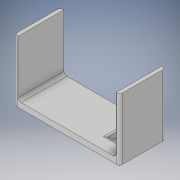
# Autodesk Inventor part: switch mount
Saved by Autodesk Inventor 2017 (Build 210142000, 142)
## iProperties
Created: 2017-11-26
Part Number: switch mount
Material: Generic
Document SubType Name: Modeling
Designer: Mitch
Density: 1 g/cm^3
Appearance: Default
Author: Mitch
Autodesk Inventor part; units mm, degrees
ref_plane "YZ Plane" through (0, 0, 0) normal (1, 0, 0) x (0, 1, 0)
ref_plane "XZ Plane" through (0, 0, 0) normal (0, 1, 0) x (-1, 0, 0)
ref_plane "XY Plane" through (0, 0, 0) normal (0, 0, 1) x (1, 0, 0)
sketch "Sketch1" plane through (0, 0, 0) normal (0, 1, 0) x (-1, 0, 0)
  line L0 (0, 0) -> (57.023, 0)
  line L1 (57.023, 0) -> (57.023, -24.765)
  line L2 (57.023, -24.765) -> (0, -24.765)
  line L3 (0, -24.765) -> (0, 0)
  dimension "d0" = 57.023
  dimension "d1" = 24.765
  constraints: 8 end point, 2 parallel, 1 horizontal, 1 perpendicular
  measures "d0" distance of L1.end L2.end
  measures "d1" distance of L0.end L1.end
extrude "Extrusion1" add sketch "Sketch1" along normal blind 3.175
sketch "Sketch3" plane through (0, 0, 0) normal (0, -1, 0) x (1, 0, 0)
  line L0 (-3.175, -3.175) -> (-15.113, -3.175)
  line L1 (-15.113, -3.175) -> (-15.113, -21.59)
  line L2 (-15.113, -21.59) -> (-3.175, -21.59)
  line L3 (-3.175, -21.59) -> (-3.175, -3.175)
  line L4 (0, -24.765) -> (0, 0) projected
  line L5 (-57.023, 0) -> (0, 0) projected
  dimension "d18" = 18.415
  dimension "d19" = 11.938
  dimension "d20" = 3.175
  dimension "d21" = 3.175
  constraints: 8 end point, 2 parallel, 1 horizontal, 1 perpendicular
  measures "d18" distance of L2.end L0.start
  measures "d19" distance of L1.end L2.end
  measures "d20" distance between parallel lines of L4 L3
  measures "d21" distance between parallel lines of L5 L0
extrude "Extrusion3" add sketch "Sketch3" along normal blind 2.921
fillet "Fillet2" radius 1.5875 4 edges at (0, 1.5875, -24.765) (0, 1.5875, 0) (-57.023, 1.5875, 0) (-57.023, 1.5875, -24.765)
hole "Hole2" at (-9.144, -2.921, -12.3825) direction (0, 1, 0) diameter 10.16 depth 25.4
sketch "Sketch4" plane through (0, 3.175, 0) normal (0, 1, 0) x (1, 0, 0)
  line L0 (-3.8735, 17.653) -> (-14.4145, 17.653)
  line L1 (-14.4145, 17.653) -> (-14.4145, 7.112)
  line L2 (-14.4145, 7.112) -> (-3.8735, 7.112)
  line L3 (-3.8735, 7.112) -> (-3.8735, 17.653)
  line L4 (-1.5875, 24.765) -> (-55.4355, 24.765) projected
  line L5 (0, 1.5875) -> (0, 23.1775) projected
  point P0 (0, 0)
  dimension "d34" = 10.541
  dimension "d35" = 10.541
  dimension "d36" = 7.112
  dimension "d37" = 3.8735
  constraints: 8 end point, 2 parallel, 1 horizontal, 1 perpendicular
  measures "d34" distance of L2.end L1.end
  measures "d35" distance of L1.end L0.end
  measures "d36" distance between parallel lines of L4 L0
  measures "d37" distance between parallel lines of L5 L3
extrude "Extrusion4" cut sketch "Sketch4" against normal blind 3.175
sketch "Sketch5" plane through (0, 3.175, 0) normal (0, 1, 0) x (1, 0, 0)
  line L0 (0, 1.5875) -> (0, 23.1775) projected
  line L1 (-1.9431, 1.5875) -> (-1.9431, 23.1775)
  line L2 (-55.4355, 24.765) -> (-1.5875, 24.765) projected
  line L3 (-1.5875, 0) -> (-1.9431, 0)
  line L4 (-1.9431, 0) -> (-1.9431, 24.765)
  line L5 (-1.9431, 24.765) -> (-1.5875, 24.765)
  line L6 (0, 23.1775) -> (0, 1.5875)
  arc A0 (0, 23.1775) -> (-1.5875, 24.765) centre (-1.5875, 23.1775) ccw
  arc A1 (-1.5875, 0) -> (0, 1.5875) centre (-1.5875, 1.5875) ccw
  line L7 (-57.023, 23.1775) -> (-57.023, 1.5875) projected
  line L8 (-55.0672, 23.1775) -> (-55.0672, 1.5875)
  line L9 (-1.5875, 0) -> (-55.4355, 0) projected
  line L10 (-55.0672, 0) -> (-55.4355, 0)
  line L11 (-57.023, 1.5875) -> (-57.023, 23.1775)
  line L12 (-55.4355, 24.765) -> (-55.0672, 24.765)
  line L13 (-55.0672, 24.765) -> (-55.0672, 0)
  arc A2 (-57.023, 1.5875) -> (-55.4355, 0) centre (-55.4355, 1.5875) ccw
  arc A3 (-55.4355, 24.765) -> (-57.023, 23.1775) centre (-55.4355, 23.1775) ccw
  point P0 (0, 0)
  dimension "d40" = 1.9431
  dimension "d41" = 1.5875
  dimension "d42" = 1.9558
  dimension "d43" = 1.5875
  constraints: 20 end point, 8 point on circle, 8 tangent, 6 parallel, 4 centre point, 4 point on line, 2 equal radius, 2 horizontal, 2 perpendicular
  measures "d40" distance between parallel lines of L0 L1
  measures "d41" radius of A0
  measures "d42" distance between parallel lines of L7 L8
  measures "d43" radius of A2
extrude "Extrusion5" add sketch "Sketch5" along normal blind 30.5308 contours A1 L3 L4 L1 L2 A0 L0 | L9 A2 L7 A3 L2 L13 L8
fillet "Fillet3" radius 1.5875 2 edges at (-1.9431, 3.175, -12.3825) (-55.0672, 3.175, -12.3825)
fillet "Fillet4" radius 0.7937 4 edges at (-9.144, 3.175, -7.112) (-14.4145, 3.175, -12.3825) (-3.8735, 3.175, -12.3825) (-9.144, 3.175, -17.653)
body "Solid1"
